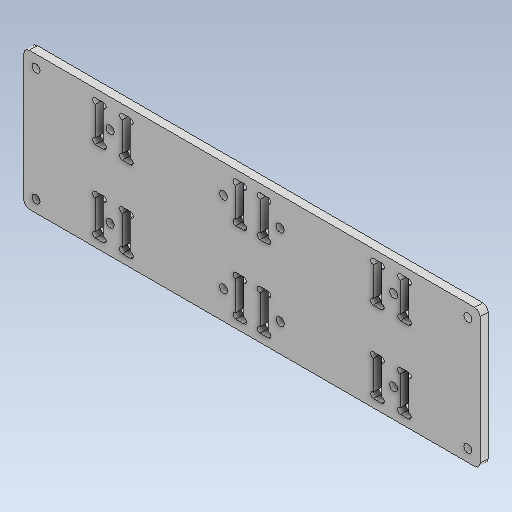
# Autodesk Inventor part: シールド板
Saved by Autodesk Inventor 2020 (Build 240168000, 168)
## iProperties
Created: 2020-02-05
Part Number: シールド板
Material: 一般
Document SubType Name: Modeling
Designer: tanjihayato
Density: 1 g/cm^3
Appearance: 既定
Mass: 23.7229 g
Surface Area: 189.328 cm^2
Volume: 23.7229 cm^3
Author: tanjihayato
Autodesk Inventor part; units mm, degrees
ref_plane "YZ Plane" through (0, 0, 0) normal (1, 0, 0) x (0, 1, 0)
ref_plane "XZ Plane" through (0, 0, 0) normal (0, 1, 0) x (-1, 0, 0)
ref_plane "XY Plane" through (0, 0, 0) normal (0, 0, 1) x (1, 0, 0)
sketch "スケッチ1" plane through (0, 0, 0) normal (0, 0, 1) x (1, 0, 0)
  line L0 (0, 0) -> (3, 0)
  line L1 (3, 0) -> (3, -15)
  line L2 (3, -15) -> (0, -15)
  line L3 (0, -15) -> (0, 0)
  line L4 (-9, 0) -> (-6, 0)
  line L5 (-6, 0) -> (-6, -15)
  line L6 (-6, -15) -> (-9, -15)
  line L7 (-9, -15) -> (-9, 0)
  line L8 (0, -30) -> (3, -30)
  line L9 (3, -30) -> (3, -45)
  line L10 (3, -45) -> (0, -45)
  line L11 (0, -45) -> (0, -30)
  line L12 (-9, -30) -> (-6, -30)
  line L13 (-6, -30) -> (-6, -45)
  line L14 (-6, -45) -> (-9, -45)
  line L15 (-9, -45) -> (-9, -30)
  line L16 (-87.5, 3) -> (81.5, 3)
  line L17 (-87.5, 3) -> (-87.5, -48)
  line L18 (-87.5, -48) -> (81.5, -48)
  line L19 (81.5, -48) -> (81.5, 3)
  circle A0 centre (-83, -1.5) radius 1.5
  circle A1 centre (77, -1.5) radius 1.5
  circle A2 centre (77, -43.5) radius 1.5
  circle A3 centre (-83, -43.5) radius 1.5
  circle A4 centre (3, -1.05) radius 1.05
  circle A5 centre (3, -13.95) radius 1.05
  circle A6 centre (0, -13.95) radius 1.05
  circle A7 centre (0, -1.05) radius 1.05
  circle A8 centre (-6, -1.05) radius 1.05
  circle A9 centre (-6, -13.95) radius 1.05
  circle A10 centre (-9, -13.95) radius 1.05
  circle A11 centre (-9, -1.05) radius 1.05
  circle A12 centre (-6, -31.05) radius 1.05
  circle A13 centre (-6, -43.95) radius 1.05
  circle A14 centre (-9, -43.95) radius 1.05
  circle A15 centre (-9, -31.05) radius 1.05
  circle A16 centre (0, -31.05) radius 1.05
  circle A17 centre (3, -31.05) radius 1.05
  circle A18 centre (3, -43.95) radius 1.05
  circle A19 centre (0, -43.95) radius 1.05
  circle A20 centre (-13.5, -7.5) radius 1.5
  circle A21 centre (7.5, -7.5) radius 1.5
  circle A22 centre (7.5, -37.5) radius 1.5
  circle A23 centre (-13.5, -37.5) radius 1.5
  line L20 (42, 0) -> (45, 0)
  line L21 (45, 0) -> (45, -15)
  line L22 (45, -15) -> (42, -15)
  line L23 (42, -15) -> (42, 0)
  line L24 (42, -30) -> (45, -30)
  line L25 (45, -30) -> (45, -45)
  line L26 (45, -45) -> (42, -45)
  line L27 (42, -45) -> (42, -30)
  circle A24 centre (45, -1.05) radius 1.05
  circle A25 centre (45, -13.95) radius 1.05
  circle A26 centre (42, -13.95) radius 1.05
  circle A27 centre (42, -1.05) radius 1.05
  circle A28 centre (42, -31.05) radius 1.05
  circle A29 centre (45, -31.05) radius 1.05
  circle A30 centre (45, -43.95) radius 1.05
  circle A31 centre (42, -43.95) radius 1.05
  circle A32 centre (49.5, -7.5) radius 1.5
  circle A33 centre (49.5, -37.5) radius 1.5
  line L28 (-51, 0) -> (-48, 0)
  line L29 (-48, 0) -> (-48, -15)
  line L30 (-48, -15) -> (-51, -15)
  line L31 (-51, -15) -> (-51, 0)
  line L32 (-51, -30) -> (-48, -30)
  line L33 (-48, -30) -> (-48, -45)
  line L34 (-48, -45) -> (-51, -45)
  line L35 (-51, -45) -> (-51, -30)
  circle A34 centre (-48, -1.05) radius 1.05
  circle A35 centre (-48, -13.95) radius 1.05
  circle A36 centre (-51, -13.95) radius 1.05
  circle A37 centre (-51, -1.05) radius 1.05
  circle A38 centre (-48, -31.05) radius 1.05
  circle A39 centre (-48, -43.95) radius 1.05
  circle A40 centre (-51, -43.95) radius 1.05
  circle A41 centre (-51, -31.05) radius 1.05
  circle A42 centre (-55.5, -7.5) radius 1.5
  circle A43 centre (-55.5, -37.5) radius 1.5
  line L36 (55, -30) -> (55, -45)
  line L37 (55, -45) -> (52, -45)
  circle A44 centre (52, -43.95) radius 1.05
  line L38 (52, -45) -> (52, -30)
  circle A45 centre (55, -43.95) radius 1.05
  line L39 (52, 0) -> (55, 0)
  line L40 (55, 0) -> (55, -15)
  line L41 (55, -15) -> (52, -15)
  line L42 (52, -15) -> (52, 0)
  circle A46 centre (55, -1.05) radius 1.05
  circle A47 centre (52, -1.05) radius 1.05
  circle A48 centre (52, -13.95) radius 1.05
  circle A49 centre (55, -13.95) radius 1.05
  line L43 (52, -30) -> (55, -30)
  circle A50 centre (55, -31.05) radius 1.05
  circle A51 centre (52, -31.05) radius 1.05
  line L44 (-61, -15) -> (-61, 0)
  line L45 (-58, -30) -> (-58, -45)
  line L46 (-61, -45) -> (-61, -30)
  line L47 (-58, 0) -> (-58, -15)
  circle A52 centre (-58, -31.05) radius 1.05
  circle A53 centre (-58, -43.95) radius 1.05
  circle A54 centre (-61, -13.95) radius 1.05
  circle A55 centre (-58, -1.05) radius 1.05
  circle A56 centre (-61, -1.05) radius 1.05
  circle A57 centre (-58, -13.95) radius 1.05
  line L48 (-58, -45) -> (-61, -45)
  line L49 (-61, -30) -> (-58, -30)
  line L50 (-61, 0) -> (-58, 0)
  line L51 (-58, -15) -> (-61, -15)
  circle A58 centre (-61, -43.95) radius 1.05
  circle A59 centre (-61, -31.05) radius 1.05
  point P0 (0, -42.9)
  point P1 (0, -32.1)
  point P2 (3, -32.1)
  point P3 (3, -42.9)
  point P4 (0, -2.1)
  point P5 (3, -2.1)
  point P6 (3, -12.9)
  point P7 (0, -12.9)
  point P8 (-9, -2.1)
  point P9 (-6, 0)
  point P10 (-6, -2.1)
  point P11 (-6, -12.9)
  point P12 (-9, -12.9)
  point P13 (-9, -32.1)
  point P14 (-6, -32.1)
  point P15 (-6, -42.9)
  point P16 (-9, -42.9)
  point P17 (-4.9275, 0)
  point P18 (1, -30)
  point P19 (-51, -32.1)
  point P20 (-48, -32.1)
  point P21 (-48, -42.9)
  point P22 (-51, -42.9)
  point P23 (42, -12.9)
  point P24 (42, -2.1)
  point P25 (45, -2.1)
  point P26 (45, -12.9)
  point P27 (42, -32.1)
  point P28 (45, -32.1)
  point P29 (45, -42.9)
  point P30 (42, -42.9)
  point P31 (-51, -12.9)
  point P32 (-51, -2.1)
  point P33 (-51, 0)
  point P34 (-48, -2.1)
  point P35 (-48, -12.9)
  point P36 (5.0725, 0)
  point P37 (11, -30)
  point P38 (-61, -42.9)
  point P39 (-61, -32.1)
  point P40 (-58, -32.1)
  point P41 (-58, -42.9)
  point P42 (-61, -2.1)
  point P43 (-61, 0)
  point P44 (-58, -2.1)
  point P45 (-58, -12.9)
  point P46 (-61, -12.9)
  point P47 (52, -42.9)
  point P48 (52, -32.1)
  point P49 (55, -32.1)
  point P50 (55, -42.9)
  point P51 (55, -2.1)
  point P52 (55, -12.9)
  point P53 (52, -12.9)
  point P54 (52, -2.1)
  dimension "d0" = 3
  dimension "d1" = 15
  dimension "d2" = 3
  dimension "d3" = 15
  dimension "d4" = 3
  dimension "d5" = 15
  dimension "d6" = 3
  dimension "d7" = 15
  dimension "d8" = 15
  dimension "d9" = 6
  dimension "d10" = 3
  dimension "d11" = 3
  dimension "d13" = 3
  dimension "d14" = 3
  dimension "d15" = 3
  dimension "d16" = 3
  dimension "d17" = 4.5
  dimension "d18" = 4.5
  dimension "d19" = 4.5
  dimension "d20" = 4.5
  dimension "d21" = 4.5
  dimension "d22" = 4.5
  dimension "d23" = 4.5
  dimension "d24" = 4.5
  dimension "d25" = 160
  dimension "d26" = 74
  dimension "d27" = 2.1
  dimension "d31" = 3
  dimension "d32" = 3
  dimension "d33" = 3
  dimension "d34" = 3
  dimension "d35" = 4.5
  dimension "d36" = 4.5
  dimension "d37" = 4.5
  dimension "d38" = 4.5
  dimension "d39" = 7.5
  dimension "d40" = 7.5
  dimension "d41" = 7.5
  dimension "d42" = 7.5
  dimension "d43" = 3
  dimension "d44" = 15
  dimension "d45" = 3
  dimension "d46" = 15
  dimension "d47" = 15
  dimension "d48" = 2.1
  dimension "d49" = 3
  dimension "d50" = 3
  dimension "d51" = 4.5
  dimension "d52" = 4.5
  dimension "d53" = 7.5
  dimension "d54" = 7.5
  dimension "d55" = 3
  dimension "d56" = 15
  dimension "d57" = 3
  dimension "d58" = 15
  dimension "d59" = 3
  dimension "d60" = 3
  dimension "d61" = 4.5
  dimension "d62" = 4.5
  dimension "d63" = 7.5
  dimension "d64" = 7.5
  dimension "d65" = 3
  dimension "d66" = 90
  dimension "d67" = 36.5
  constraints: 104 end point, 60 centre point, 60 point on line, 48 tangent, 43 equal radius, 24 parallel, 14 perpendicular, 13 horizontal, 2 collinear, 1 vertical
  measures "d0" distance of L1.end L2.end
  measures "d1" distance of L0.end L1.end
  measures "d2" distance of L5.end L6.end
  measures "d3" distance of L4.end L5.end
  measures "d4" distance of L9.end L10.end
  measures "d5" distance of L8.end L9.end
  measures "d6" distance of L13.end L14.end
  measures "d7" distance of L12.end L13.end
  measures "d8" distance between parallel lines of L8 L2
  measures "d9" distance between parallel lines of L13 L11
  measures "d10" distance between parallel lines of L4 L16
  measures "d11" distance between parallel lines of L18 L10
  measures "d13" diameter of A0
  measures "d14" diameter of A1
  measures "d15" diameter of A2
  measures "d16" diameter of A3
  measures "d17" distance from line of A0.centre L16
  measures "d18" distance from line of L17 A0.centre
  measures "d19" distance from line of L18 A3.centre
  measures "d20" distance from line of L17 A3.centre
  measures "d21" distance from line of L18 A2.centre
  measures "d22" distance from line of L19 A2.centre
  measures "d23" distance from line of L19 A1.centre
  measures "d24" distance from line of L16 A1.centre
  measures "d25" distance of A1.centre A0.centre
  measures "d26" distance from line of L1 A1.centre
  measures "d27" diameter of A4
  measures "d31" diameter of A20
  measures "d32" diameter of A21
  measures "d33" diameter of A22
  measures "d34" diameter of A23
  measures "d35" distance from line of A20.centre L7
  measures "d36" distance from line of L1 A21.centre
  measures "d37" distance from line of L9 A22.centre
  measures "d38" distance from line of L15 A23.centre
  measures "d39" distance from line of A21.centre L0
  measures "d40" distance from line of A20.centre L4
  measures "d41" distance from line of L14 A23.centre
  measures "d42" distance from line of L10 A22.centre
  measures "d43" distance of L21.end L22.end
  measures "d44" distance of L20.end L21.end
  measures "d45" distance of L25.end L26.end
  measures "d46" distance of L25.start L25.end
  measures "d47" distance between parallel lines of L24 L22
  measures "d48" diameter of A24
  measures "d49" diameter of A32
  measures "d50" diameter of A33
  measures "d51" distance from line of L21 A32.centre
  measures "d52" distance from line of L25 A33.centre
  measures "d53" distance from line of A32.centre L20
  measures "d54" distance from line of L26 A33.centre
  measures "d55" distance of L29.end L31.start
  measures "d56" distance of L29.start L29.end
  measures "d57" distance of L33.end L35.start
  measures "d58" distance of L33.start L33.end
  measures "d59" diameter of A42
  measures "d60" diameter of A43
  measures "d61" distance from line of A42.centre L31
  measures "d62" distance from line of L35 A43.centre
  measures "d63" distance from line of A42.centre L28
  measures "d64" distance from line of L34 A43.centre
  measures "d65" distance between parallel lines of L18 L26
  measures "d66" distance between parallel lines of L23 L29
  measures "d67" distance between parallel lines of L19 L21
extrude "押し出し1" add sketch "スケッチ1" along normal blind 3
fillet "フィレット1" radius 2 4 edges at (81.5, 3, 1.5) (81.5, -48, 1.5) (-87.5, -48, 1.5) (-87.5, 3, 1.5)
